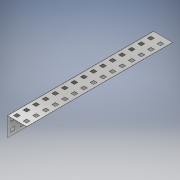
# Autodesk Inventor part: 2sqr x 2sqr metal frame
Saved by Autodesk Inventor 2018 (Build 220112000, 112)
## iProperties
Created: 2018-10-16
Part Number: 2sqr x 2sqr metal frame
Material: Generic
Document SubType Name: Modeling
Designer: USER
Density: 1 g/cm^3
Appearance: Machined - Aluminum
Author: USER
Autodesk Inventor part; units mm, degrees
ref_plane "YZ Plane" through (0, 0, 0) normal (1, 0, 0) x (0, 1, 0)
ref_plane "XZ Plane" through (0, 0, 0) normal (0, 1, 0) x (-1, 0, 0)
ref_plane "XY Plane" through (0, 0, 0) normal (0, 0, 1) x (1, 0, 0)
sketch "Sketch1" plane through (0, 0, 0) normal (1, 0, 0) x (0, 1, 0)
  line L0 (0, 0) -> (-24.9936, 0)
  line L1 (-24.9936, 0) -> (-24.9936, -189.992)
  line L2 (-24.9936, -189.992) -> (0, -189.992)
  line L3 (0, -189.992) -> (0, 0)
  dimension "d0" = 24.9936
  dimension "d1" = 189.992
  constraints: 8 end point, 2 parallel, 1 horizontal, 1 perpendicular
  measures "d0" distance of L2.end L1.end
  measures "d1" distance of L1.end L0.end
sketch "Sketch2" plane through (0, 0, 0) normal (0, 1, 0) x (-1, 0, 0)
  line L0 (0, 0) -> (-24.9936, 0)
  line L1 (-24.9936, 0) -> (-24.9936, -189.992)
  line L2 (-24.9936, -189.992) -> (0, -189.992)
  line L3 (0, -189.992) -> (0, 0)
  dimension "d2" = 24.9936
  dimension "d3" = 189.992
  constraints: 8 end point, 2 parallel, 1 horizontal, 1 perpendicular
  measures "d2" distance of L2.end L1.end
  measures "d3" distance of L1.end L0.end
extrude "Extrusion1" add sketch "Sketch2" against normal blind 0.254
extrude "Extrusion2" add sketch "Sketch1" along normal blind 0.254 separate body
sketch "Sketch3" plane through (0, 0, 0) normal (0, 1, 0) x (1, 0, 0)
  line L0 (21.082, 3.9116) -> (16.51, 3.9116)
  line L1 (16.51, 3.9116) -> (16.51, 8.4836)
  line L2 (16.51, 8.4836) -> (21.082, 8.4836)
  line L3 (21.082, 8.4836) -> (21.082, 3.9116)
  line L4 (24.9936, 0) -> (24.9936, 189.992) projected
  line L5 (16.51, 20.9296) -> (21.082, 20.9296)
  line L6 (21.082, 20.9296) -> (21.082, 16.3576)
  line L7 (21.082, 16.3576) -> (16.51, 16.3576)
  line L8 (16.51, 16.3576) -> (16.51, 20.9296)
  line L9 (16.51, 33.3756) -> (21.082, 33.3756)
  line L10 (21.082, 33.3756) -> (21.082, 28.8036)
  line L11 (21.082, 28.8036) -> (16.51, 28.8036)
  line L12 (16.51, 28.8036) -> (16.51, 33.3756)
  line L13 (16.51, 45.8216) -> (21.082, 45.8216)
  line L14 (21.082, 45.8216) -> (21.082, 41.2496)
  line L15 (21.082, 41.2496) -> (16.51, 41.2496)
  line L16 (16.51, 41.2496) -> (16.51, 45.8216)
  line L17 (16.51, 58.2676) -> (21.082, 58.2676)
  line L18 (21.082, 58.2676) -> (21.082, 53.6956)
  line L19 (21.082, 53.6956) -> (16.51, 53.6956)
  line L20 (16.51, 53.6956) -> (16.51, 58.2676)
  line L21 (16.51, 70.7136) -> (21.082, 70.7136)
  line L22 (21.082, 70.7136) -> (21.082, 66.1416)
  line L23 (21.082, 66.1416) -> (16.51, 66.1416)
  line L24 (16.51, 66.1416) -> (16.51, 70.7136)
  line L25 (16.51, 83.1596) -> (21.082, 83.1596)
  line L26 (21.082, 83.1596) -> (21.082, 78.5876)
  line L27 (21.082, 78.5876) -> (16.51, 78.5876)
  line L28 (16.51, 78.5876) -> (16.51, 83.1596)
  line L29 (16.51, 95.6056) -> (21.082, 95.6056)
  line L30 (21.082, 95.6056) -> (21.082, 91.0336)
  line L31 (21.082, 91.0336) -> (16.51, 91.0336)
  line L32 (16.51, 91.0336) -> (16.51, 95.6056)
  line L33 (16.51, 108.0516) -> (21.082, 108.0516)
  line L34 (21.082, 108.0516) -> (21.082, 103.4796)
  line L35 (21.082, 103.4796) -> (16.51, 103.4796)
  line L36 (16.51, 103.4796) -> (16.51, 108.0516)
  line L37 (16.51, 120.4976) -> (21.082, 120.4976)
  line L38 (21.082, 120.4976) -> (21.082, 115.9256)
  line L39 (21.082, 115.9256) -> (16.51, 115.9256)
  line L40 (16.51, 115.9256) -> (16.51, 120.4976)
  line L41 (16.51, 132.9436) -> (21.082, 132.9436)
  line L42 (21.082, 132.9436) -> (21.082, 128.3716)
  line L43 (21.082, 128.3716) -> (16.51, 128.3716)
  line L44 (16.51, 128.3716) -> (16.51, 132.9436)
  line L45 (16.51, 145.3896) -> (21.082, 145.3896)
  line L46 (21.082, 145.3896) -> (21.082, 140.8176)
  line L47 (21.082, 140.8176) -> (16.51, 140.8176)
  line L48 (16.51, 140.8176) -> (16.51, 145.3896)
  line L49 (16.51, 157.8356) -> (21.082, 157.8356)
  line L50 (21.082, 157.8356) -> (21.082, 153.2636)
  line L51 (21.082, 153.2636) -> (16.51, 153.2636)
  line L52 (16.51, 153.2636) -> (16.51, 157.8356)
  line L53 (16.51, 170.2816) -> (21.082, 170.2816)
  line L54 (21.082, 170.2816) -> (21.082, 165.7096)
  line L55 (21.082, 165.7096) -> (16.51, 165.7096)
  line L56 (16.51, 165.7096) -> (16.51, 170.2816)
  line L57 (16.51, 182.7276) -> (21.082, 182.7276)
  line L58 (21.082, 182.7276) -> (21.082, 178.1556)
  line L59 (21.082, 178.1556) -> (16.51, 178.1556)
  line L60 (16.51, 178.1556) -> (16.51, 182.7276)
  line L61 (0, 189.992) -> (24.9936, 189.992) projected
  line L62 (24.9936, 0) -> (0, 0) projected
  line L63 (3.9116, 3.9116) -> (8.4836, 3.9116)
  line L64 (8.4836, 3.9116) -> (8.4836, 8.4836)
  line L65 (8.4836, 8.4836) -> (3.9116, 8.4836)
  line L66 (3.9116, 8.4836) -> (3.9116, 3.9116)
  line L67 (8.4836, 20.9296) -> (3.9116, 20.9296)
  line L68 (3.9116, 20.9296) -> (3.9116, 16.3576)
  line L69 (3.9116, 16.3576) -> (8.4836, 16.3576)
  line L70 (8.4836, 16.3576) -> (8.4836, 20.9296)
  line L71 (8.4836, 33.3756) -> (3.9116, 33.3756)
  line L72 (3.9116, 33.3756) -> (3.9116, 28.8036)
  line L73 (3.9116, 28.8036) -> (8.4836, 28.8036)
  line L74 (8.4836, 28.8036) -> (8.4836, 33.3756)
  line L75 (8.4836, 45.8216) -> (3.9116, 45.8216)
  line L76 (3.9116, 45.8216) -> (3.9116, 41.2496)
  line L77 (3.9116, 41.2496) -> (8.4836, 41.2496)
  line L78 (8.4836, 41.2496) -> (8.4836, 45.8216)
  line L79 (8.4836, 58.2676) -> (3.9116, 58.2676)
  line L80 (3.9116, 58.2676) -> (3.9116, 53.6956)
  line L81 (3.9116, 53.6956) -> (8.4836, 53.6956)
  line L82 (8.4836, 53.6956) -> (8.4836, 58.2676)
  line L83 (8.4836, 70.7136) -> (3.9116, 70.7136)
  line L84 (3.9116, 70.7136) -> (3.9116, 66.1416)
  line L85 (3.9116, 66.1416) -> (8.4836, 66.1416)
  line L86 (8.4836, 66.1416) -> (8.4836, 70.7136)
  line L87 (8.4836, 83.1596) -> (3.9116, 83.1596)
  line L88 (3.9116, 83.1596) -> (3.9116, 78.5876)
  line L89 (3.9116, 78.5876) -> (8.4836, 78.5876)
  line L90 (8.4836, 78.5876) -> (8.4836, 83.1596)
  line L91 (8.4836, 95.6056) -> (3.9116, 95.6056)
  line L92 (3.9116, 95.6056) -> (3.9116, 91.0336)
  line L93 (3.9116, 91.0336) -> (8.4836, 91.0336)
  line L94 (8.4836, 91.0336) -> (8.4836, 95.6056)
  line L95 (8.4836, 108.0516) -> (3.9116, 108.0516)
  line L96 (3.9116, 108.0516) -> (3.9116, 103.4796)
  line L97 (3.9116, 103.4796) -> (8.4836, 103.4796)
  line L98 (8.4836, 103.4796) -> (8.4836, 108.0516)
  line L99 (8.4836, 120.4976) -> (3.9116, 120.4976)
  line L100 (3.9116, 120.4976) -> (3.9116, 115.9256)
  line L101 (3.9116, 115.9256) -> (8.4836, 115.9256)
  line L102 (8.4836, 115.9256) -> (8.4836, 120.4976)
  line L103 (8.4836, 132.9436) -> (3.9116, 132.9436)
  line L104 (3.9116, 132.9436) -> (3.9116, 128.3716)
  line L105 (3.9116, 128.3716) -> (8.4836, 128.3716)
  line L106 (8.4836, 128.3716) -> (8.4836, 132.9436)
  line L107 (8.4836, 145.3896) -> (3.9116, 145.3896)
  line L108 (3.9116, 145.3896) -> (3.9116, 140.8176)
  line L109 (3.9116, 140.8176) -> (8.4836, 140.8176)
  line L110 (8.4836, 140.8176) -> (8.4836, 145.3896)
  line L111 (8.4836, 157.8356) -> (3.9116, 157.8356)
  line L112 (3.9116, 157.8356) -> (3.9116, 153.2636)
  line L113 (3.9116, 153.2636) -> (8.4836, 153.2636)
  line L114 (8.4836, 153.2636) -> (8.4836, 157.8356)
  line L115 (8.4836, 170.2816) -> (3.9116, 170.2816)
  line L116 (3.9116, 170.2816) -> (3.9116, 165.7096)
  line L117 (3.9116, 165.7096) -> (8.4836, 165.7096)
  line L118 (8.4836, 165.7096) -> (8.4836, 170.2816)
  line L119 (8.4836, 182.7276) -> (3.9116, 182.7276)
  line L120 (3.9116, 182.7276) -> (3.9116, 178.1556)
  line L121 (3.9116, 178.1556) -> (8.4836, 178.1556)
  line L122 (8.4836, 178.1556) -> (8.4836, 182.7276)
  dimension "d8" = 4.572
  dimension "d9" = 4.572
  dimension "d10" = 3.9116
  dimension "d16" = 12.446
  constraints: 240 end point, 2 parallel, 1 collinear, 1 horizontal, 1 perpendicular, 1 vertical, 111 other
  measures "d8" distance of L1.end L2.end
  measures "d9" distance of L0.end L1.end
  measures "d10" distance between parallel lines of L4 L3
  measures "d16" distance of L1.end L5.start
extrude "Extrusion3" cut sketch "Sketch3" against normal through all bodies 1
sketch "Sketch4" plane through (0, 0, 0) normal (-1, 0, 0) x (0, 0, 1)
  line L0 (-4.0386, -4.0386) -> (-8.6106, -4.0386)
  line L1 (-8.6106, -4.0386) -> (-8.6106, -8.6106)
  line L2 (-8.6106, -8.6106) -> (-4.0386, -8.6106)
  line L3 (-4.0386, -8.6106) -> (-4.0386, -4.0386)
  line L4 (-16.4846, -4.0386) -> (-21.0566, -4.0386)
  line L5 (-21.0566, -4.0386) -> (-21.0566, -8.6106)
  line L6 (-16.4846, -8.6106) -> (-16.4846, -4.0386)
  line L7 (-21.0566, -8.6106) -> (-16.4846, -8.6106)
  line L8 (-28.9306, -4.0386) -> (-33.5026, -4.0386)
  line L9 (-33.5026, -4.0386) -> (-33.5026, -8.6106)
  line L10 (-28.9306, -8.6106) -> (-28.9306, -4.0386)
  line L11 (-33.5026, -8.6106) -> (-28.9306, -8.6106)
  line L12 (-41.3766, -4.0386) -> (-45.9486, -4.0386)
  line L13 (-45.9486, -4.0386) -> (-45.9486, -8.6106)
  line L14 (-41.3766, -8.6106) -> (-41.3766, -4.0386)
  line L15 (-45.9486, -8.6106) -> (-41.3766, -8.6106)
  line L16 (-53.8226, -4.0386) -> (-58.3946, -4.0386)
  line L17 (-58.3946, -4.0386) -> (-58.3946, -8.6106)
  line L18 (-53.8226, -8.6106) -> (-53.8226, -4.0386)
  line L19 (-58.3946, -8.6106) -> (-53.8226, -8.6106)
  line L20 (-66.2686, -4.0386) -> (-70.8406, -4.0386)
  line L21 (-70.8406, -4.0386) -> (-70.8406, -8.6106)
  line L22 (-66.2686, -8.6106) -> (-66.2686, -4.0386)
  line L23 (-70.8406, -8.6106) -> (-66.2686, -8.6106)
  line L24 (-78.7146, -4.0386) -> (-83.2866, -4.0386)
  line L25 (-83.2866, -4.0386) -> (-83.2866, -8.6106)
  line L26 (-78.7146, -8.6106) -> (-78.7146, -4.0386)
  line L27 (-83.2866, -8.6106) -> (-78.7146, -8.6106)
  line L28 (-91.1606, -4.0386) -> (-95.7326, -4.0386)
  line L29 (-95.7326, -4.0386) -> (-95.7326, -8.6106)
  line L30 (-91.1606, -8.6106) -> (-91.1606, -4.0386)
  line L31 (-95.7326, -8.6106) -> (-91.1606, -8.6106)
  line L32 (-103.6066, -4.0386) -> (-108.1786, -4.0386)
  line L33 (-108.1786, -4.0386) -> (-108.1786, -8.6106)
  line L34 (-103.6066, -8.6106) -> (-103.6066, -4.0386)
  line L35 (-108.1786, -8.6106) -> (-103.6066, -8.6106)
  line L36 (-116.0526, -4.0386) -> (-120.6246, -4.0386)
  line L37 (-120.6246, -4.0386) -> (-120.6246, -8.6106)
  line L38 (-116.0526, -8.6106) -> (-116.0526, -4.0386)
  line L39 (-120.6246, -8.6106) -> (-116.0526, -8.6106)
  line L40 (-128.4986, -4.0386) -> (-133.0706, -4.0386)
  line L41 (-133.0706, -4.0386) -> (-133.0706, -8.6106)
  line L42 (-128.4986, -8.6106) -> (-128.4986, -4.0386)
  line L43 (-133.0706, -8.6106) -> (-128.4986, -8.6106)
  line L44 (-140.9446, -4.0386) -> (-145.5166, -4.0386)
  line L45 (-145.5166, -4.0386) -> (-145.5166, -8.6106)
  line L46 (-140.9446, -8.6106) -> (-140.9446, -4.0386)
  line L47 (-145.5166, -8.6106) -> (-140.9446, -8.6106)
  line L48 (-153.3906, -4.0386) -> (-157.9626, -4.0386)
  line L49 (-157.9626, -4.0386) -> (-157.9626, -8.6106)
  line L50 (-153.3906, -8.6106) -> (-153.3906, -4.0386)
  line L51 (-157.9626, -8.6106) -> (-153.3906, -8.6106)
  line L52 (-165.8366, -4.0386) -> (-170.4086, -4.0386)
  line L53 (-170.4086, -4.0386) -> (-170.4086, -8.6106)
  line L54 (-165.8366, -8.6106) -> (-165.8366, -4.0386)
  line L55 (-170.4086, -8.6106) -> (-165.8366, -8.6106)
  line L56 (-178.2826, -4.0386) -> (-182.8546, -4.0386)
  line L57 (-182.8546, -4.0386) -> (-182.8546, -8.6106)
  line L58 (-178.2826, -8.6106) -> (-178.2826, -4.0386)
  line L59 (-182.8546, -8.6106) -> (-178.2826, -8.6106)
  line L60 (-189.992, -24.9936) -> (-189.992, 0) projected
  line L61 (0, 0) -> (0, -24.9936) projected
  line L62 (-4.0386, -20.955) -> (-8.6106, -20.955)
  line L63 (-8.6106, -20.955) -> (-8.6106, -16.383)
  line L64 (-8.6106, -16.383) -> (-4.0386, -16.383)
  line L65 (-4.0386, -16.383) -> (-4.0386, -20.955)
  line L66 (-16.4846, -20.955) -> (-21.0566, -20.955)
  line L67 (-21.0566, -20.955) -> (-21.0566, -16.383)
  line L68 (-16.4846, -16.383) -> (-16.4846, -20.955)
  line L69 (-21.0566, -16.383) -> (-16.4846, -16.383)
  line L70 (-28.9306, -20.955) -> (-33.5026, -20.955)
  line L71 (-33.5026, -20.955) -> (-33.5026, -16.383)
  line L72 (-28.9306, -16.383) -> (-28.9306, -20.955)
  line L73 (-33.5026, -16.383) -> (-28.9306, -16.383)
  line L74 (-41.3766, -20.955) -> (-45.9486, -20.955)
  line L75 (-45.9486, -20.955) -> (-45.9486, -16.383)
  line L76 (-41.3766, -16.383) -> (-41.3766, -20.955)
  line L77 (-45.9486, -16.383) -> (-41.3766, -16.383)
  line L78 (-53.8226, -20.955) -> (-58.3946, -20.955)
  line L79 (-58.3946, -20.955) -> (-58.3946, -16.383)
  line L80 (-53.8226, -16.383) -> (-53.8226, -20.955)
  line L81 (-58.3946, -16.383) -> (-53.8226, -16.383)
  line L82 (-66.2686, -20.955) -> (-70.8406, -20.955)
  line L83 (-70.8406, -20.955) -> (-70.8406, -16.383)
  line L84 (-66.2686, -16.383) -> (-66.2686, -20.955)
  line L85 (-70.8406, -16.383) -> (-66.2686, -16.383)
  line L86 (-78.7146, -20.955) -> (-83.2866, -20.955)
  line L87 (-83.2866, -20.955) -> (-83.2866, -16.383)
  line L88 (-78.7146, -16.383) -> (-78.7146, -20.955)
  line L89 (-83.2866, -16.383) -> (-78.7146, -16.383)
  line L90 (-91.1606, -20.955) -> (-95.7326, -20.955)
  line L91 (-95.7326, -20.955) -> (-95.7326, -16.383)
  line L92 (-91.1606, -16.383) -> (-91.1606, -20.955)
  line L93 (-95.7326, -16.383) -> (-91.1606, -16.383)
  line L94 (-103.6066, -20.955) -> (-108.1786, -20.955)
  line L95 (-108.1786, -20.955) -> (-108.1786, -16.383)
  line L96 (-103.6066, -16.383) -> (-103.6066, -20.955)
  line L97 (-108.1786, -16.383) -> (-103.6066, -16.383)
  line L98 (-116.0526, -20.955) -> (-120.6246, -20.955)
  line L99 (-120.6246, -20.955) -> (-120.6246, -16.383)
  line L100 (-116.0526, -16.383) -> (-116.0526, -20.955)
  line L101 (-120.6246, -16.383) -> (-116.0526, -16.383)
  line L102 (-128.4986, -20.955) -> (-133.0706, -20.955)
  line L103 (-133.0706, -20.955) -> (-133.0706, -16.383)
  line L104 (-128.4986, -16.383) -> (-128.4986, -20.955)
  line L105 (-133.0706, -16.383) -> (-128.4986, -16.383)
  line L106 (-140.9446, -20.955) -> (-145.5166, -20.955)
  line L107 (-145.5166, -20.955) -> (-145.5166, -16.383)
  line L108 (-140.9446, -16.383) -> (-140.9446, -20.955)
  line L109 (-145.5166, -16.383) -> (-140.9446, -16.383)
  line L110 (-153.3906, -20.955) -> (-157.9626, -20.955)
  line L111 (-157.9626, -20.955) -> (-157.9626, -16.383)
  line L112 (-153.3906, -16.383) -> (-153.3906, -20.955)
  line L113 (-157.9626, -16.383) -> (-153.3906, -16.383)
  line L114 (-165.8366, -20.955) -> (-170.4086, -20.955)
  line L115 (-170.4086, -20.955) -> (-170.4086, -16.383)
  line L116 (-165.8366, -16.383) -> (-165.8366, -20.955)
  line L117 (-170.4086, -16.383) -> (-165.8366, -16.383)
  line L118 (-178.2826, -20.955) -> (-182.8546, -20.955)
  line L119 (-182.8546, -20.955) -> (-182.8546, -16.383)
  line L120 (-178.2826, -16.383) -> (-178.2826, -20.955)
  line L121 (-182.8546, -16.383) -> (-178.2826, -16.383)
  dimension "d20" = 4.572
  dimension "d21" = 4.572
  dimension "d27" = 12.446
  constraints: 240 end point, 2 horizontal, 2 parallel, 1 collinear, 1 perpendicular, 111 other
  measures "d20" distance of L2.end L1.end
  measures "d21" distance of L1.end L0.end
  measures "d27" distance of L0.start L4.start
extrude "Extrusion4" cut sketch "Sketch4" against normal through all bodies 2
body "Solid1"
body "Solid2"
